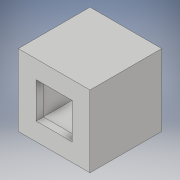
# Autodesk Inventor part: secondary_part
Saved by Autodesk Inventor 2019 (Build 230136000, 136)
## iProperties
Created: 2019-02-05
Part Number: secondary_part
Material: Generic
Document SubType Name: Modeling
Designer: ybharatu
Density: 1 g/cm^3
Appearance: Default
Author: ybharatu
Autodesk Inventor part; units mm, degrees
ref_plane "YZ Plane" through (0, 0, 0) normal (1, 0, 0) x (0, 1, 0)
ref_plane "XZ Plane" through (0, 0, 0) normal (0, 1, 0) x (-1, 0, 0)
ref_plane "XY Plane" through (0, 0, 0) normal (0, 0, 1) x (1, 0, 0)
sketch "Sketch1" plane through (0, 0, 0) normal (0, 0, 1) x (1, 0, 0)
  line L0 (-24.3417, 44.0972) -> (51.8583, 44.0972)
  line L1 (51.8583, 44.0972) -> (51.8583, -32.1028)
  line L2 (51.8583, -32.1028) -> (-24.3417, -32.1028)
  line L3 (-24.3417, -32.1028) -> (-24.3417, 44.0972)
  point P0 (0, 0)
  dimension "d0" = 76.2
  dimension "d1" = 76.2
  constraints: 8 end point, 2 parallel, 1 horizontal, 1 perpendicular
  measures "d0" distance of L0.end L1.end
  measures "d1" distance of L0.start L0.end
extrude "Extrusion1" add sketch "Sketch1" along normal blind 76.2
shell "Shell1" thickness 7.62 removed faces 1 at (1.0583, 18.6972, 0)
sketch "Sketch2" plane through (0, 0, 76.2) normal (0, 0, 1) x (1, 0, 0)
  line L0 (-5.2917, 25.0472) -> (32.8083, 25.0472)
  line L1 (32.8083, 25.0472) -> (32.8083, -13.0528)
  line L2 (32.8083, -13.0528) -> (-5.2917, -13.0528)
  line L3 (-5.2917, -13.0528) -> (-5.2917, 25.0472)
  line L4 (51.8583, 44.0972) -> (-24.3417, 44.0972) projected
  line L5 (51.8583, -32.1028) -> (51.8583, 44.0972) projected
  point P0 (0, 0)
  dimension "d5" = 38.1
  dimension "d6" = 38.1
  dimension "d7" = 19.05
  dimension "d8" = 19.05
  constraints: 8 end point, 2 parallel, 1 horizontal, 1 perpendicular
  measures "d5" distance of L0.start L0.end
  measures "d6" distance of L2.end L0.start
  measures "d7" distance between parallel lines of L4 L0
  measures "d8" distance between parallel lines of L5 L1
extrude "Extrusion2" cut sketch "Sketch2" against normal blind 25.4
body "Solid1"
